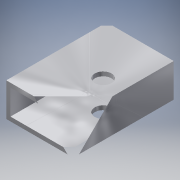
# Autodesk Inventor part: wheel arm support
Saved by Autodesk Inventor 2016 (Build 200138000, 138)
## iProperties
Created: 2016-01-17
Part Number: wheel arm support
Material: Aluminum 6061
Document SubType Name: Modeling
Designer: gus
Mass: 80.2603 g
Surface Area: 201.822 cm^2
Volume: 29.7261 cm^3
Density: 2.7 g/cm^3
Appearance: Aluminum - Flat
User Status: not complete
Author: gus
Autodesk Inventor part; units mm, degrees
ref_plane "YZ Plane" through (0, 0, 0) normal (1, 0, 0) x (0, 1, 0)
ref_plane "XZ Plane" through (0, 0, 0) normal (0, 1, 0) x (-1, 0, 0)
ref_plane "XY Plane" through (0, 0, 0) normal (0, 0, 1) x (1, 0, 0)
sketch "Sketch1" plane through (0, 0, 0) normal (0, 0, 1) x (1, 0, 0)
  line L0 (0, 0) -> (50.8, 0)
  line L1 (50.8, 0) -> (50.8, 25.4)
  line L2 (50.8, 25.4) -> (0, 25.4)
  line L3 (0, 25.4) -> (0, 0)
  line L4 (3.175, 22.225) -> (47.625, 22.225)
  line L5 (47.625, 22.225) -> (47.625, 3.175)
  line L6 (47.625, 3.175) -> (3.175, 3.175)
  line L7 (3.175, 3.175) -> (3.175, 22.225)
  dimension "d0" = 50.8
  dimension "d1" = 25.4
  dimension "d2" = 3.175
  constraints: 16 end point, 4 parallel, 2 perpendicular, 1 horizontal, 3 other
  measures "d0" distance of L2.end L1.end
  measures "d1" distance of L1.end L0.end
  measures "d2" distance between parallel lines of L2 L4
extrude "Extrusion1" add sketch "Sketch1" along normal blind 76.2
sketch "Sketch2" plane through (0, 0, 0) normal (0, -1, 0) x (1, 0, 0)
  line L0 (50.8, 0) -> (50.8, 76.2) projected
  line L1 (0, 76.2) -> (50.8, 76.2) projected
  line L2 (0, 0) -> (0, 76.2) projected
  point P0 (25.4, 38.1)
  dimension "d6" = 38.1
  dimension "d14" = 25.4
  measures "d6" distance from line of L1 point (25.4, 38.1)
  measures "d14" distance from line of point (25.4, 38.1) L2
hole "Hole1" at (25.4, 0, 38.1) direction (0, 1, 0) diameter 28.575 end through all
body "Solid1"
